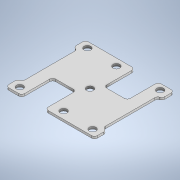
# Autodesk Inventor part: Separador engrenagens
Saved by Autodesk Inventor 2021 (Build 250183000, 183)
## iProperties
Created: 2022-03-26
Part Number: Separador engrenagens
Material: Generic
Document SubType Name: Modeling
Designer: Matheus
Density: 1.04769 g/cm^3
Appearance: Default
Mass: 3.4 g
Surface Area: 49.2715 cm^2
Volume: 3.24524 cm^3
Author: Matheus
Autodesk Inventor part; units mm, degrees
ref_plane "YZ Plane" through (0, 0, 0) normal (1, 0, 0) x (0, 1, 0)
ref_plane "XZ Plane" through (0, 0, 0) normal (0, 1, 0) x (-1, 0, 0)
ref_plane "XY Plane" through (0, 0, 0) normal (0, 0, 1) x (1, 0, 0)
sketch "Sketch1" plane through (0, 0, 0) normal (0, 1, 0) x (-1, 0, 0)
  line L0 (-29.5, 26.5) -> (29.5, 26.5)
  line L1 (29.5, 26.5) -> (29.5, -26.5)
  line L2 (29.5, -26.5) -> (-29.5, -26.5)
  line L3 (-29.5, -26.5) -> (-29.5, 26.5)
  line L4 (-29.5, 26.5) -> (29.5, -26.5) construction
  line L5 (29.5, 26.5) -> (-29.5, -26.5) construction
  point P0 (0, 0)
  dimension "d0" = 59
  dimension "d1" = 53
  constraints: 12 end point, 2 midpoint, 2 parallel, 1 horizontal, 1 perpendicular
  measures "d0" distance of L1.end L2.end
  measures "d1" distance of L0.end L1.end
extrude "Extrusion1" add sketch "Sketch1" along normal blind 1.5
sketch "Sketch2" plane through (0, 1.5, 0) normal (0, 1, 0) x (1, 0, 0)
  line L0 (41.3, 0) -> (-41.3, 0) construction
  line L1 (0, 37.1) -> (0, -37.1) construction
  line L2 (-29.5, 26.5) -> (-29.5, -26.5) construction
  point P0 (0, 0)
  point P1 (-24.25, -22.5)
  point P2 (-24.25, 22.5)
  point P3 (4.15, -21.724)
  point P4 (0, 0)
  point P5 (-4.15, 21.724)
  point P6 (24.25, -22.5)
  point P7 (24.25, 22.5)
  dimension "d5" = 21.724
  dimension "d7" = 45
  dimension "d8" = 24.25
  dimension "d9" = 21.724
  dimension "d19" = 4.15
  dimension "d20" = 4.15
  constraints: 3 symmetric about line, 1 coincident
  measures "d5" distance from line of L0 point (4.15, -21.724)
  measures "d7" distance of point (-24.25, 22.5) point (-24.25, -22.5)
  measures "d8" distance from line of L1 point (-24.25, 22.5)
  measures "d9" vertical distance of point (-4.15, 21.724) point (0, 0)
  measures "d19" distance from line of L1 point (-4.15, 21.724)
  measures "d20" distance from line of L1 point (4.15, -21.724)
hole "Hole1" at (-24.25, 1.5, 22.5) at (-24.25, 1.5, -22.5) at (4.15, 1.5, 21.724) at (0, 1.5, 0) at (-4.15, 1.5, -21.724) at (24.25, 1.5, 22.5) at (24.25, 1.5, -22.5) direction (0, -1, 0) diameter 4.5 depth 1.5
sketch "Sketch3" plane through (0, 1.5, 0) normal (0, 1, 0) x (1, 0, 0)
  line L0 (-41.3, 0) -> (41.3, 0) construction
  line L1 (0, 37.1) -> (0, -37.1) construction
  line L2 (-3.35, -26.5) -> (-19, -26.5)
  line L3 (-19, -26.5) -> (-19, -5.85)
  line L4 (-19, -5.85) -> (-3.35, -5.85)
  line L5 (-3.35, -5.85) -> (-3.35, -26.5)
  line L6 (3.35, 5.85) -> (19, 5.85)
  line L7 (19, 5.85) -> (19, 26.5)
  line L8 (19, 26.5) -> (3.35, 26.5)
  line L9 (3.35, 26.5) -> (3.35, 5.85)
  circle A0 centre (4.15, -21.724) radius 2.25 construction
  line L10 (-29.5, -26.5) -> (29.5, -26.5) construction
  circle A1 centre (-24.25, -22.5) radius 2.25 construction
  line L11 (29.5, 26.5) -> (-29.5, 26.5) construction
  circle A2 centre (24.25, 22.5) radius 2.25 construction
  circle A3 centre (-4.15, 21.724) radius 2.25 construction
  point P0 (0, 0)
  point P1 (-28.5, -26.5)
  point P2 (28.5, -26.5)
  point P3 (28.5, 26.5)
  point P4 (-28.5, 26.5)
  dimension "d21" = 7.5
  dimension "d23" = 5.25
  dimension "d24" = 20.65
  dimension "d25" = 20.65
  dimension "d26" = 7.5
  dimension "d27" = 5.25
  constraints: 16 end point, 4 parallel, 2 collinear, 2 horizontal, 2 perpendicular
  measures "d21" distance from line of L5 A0.centre
  measures "d23" distance from line of L3 A1.centre
  measures "d24" distance between parallel lines of L2 L4
  measures "d25" distance between parallel lines of L6 L8
  measures "d26" distance from line of L9 A3.centre
  measures "d27" distance from line of A2.centre L7
extrude "Extrusion2" cut sketch "Sketch3" against normal up to next
sketch "Sketch5" plane through (0, 1.5, 0) normal (0, 1, 0) x (1, 0, 0)
  line L0 (29.5, -26.5) -> (29.5, 26.5) construction
  line L1 (29.5, 18.5) -> (26.75, 18.5)
  line L2 (26.75, 18.5) -> (26.75, -18.5)
  line L3 (26.75, -18.5) -> (29.5, -18.5)
  line L4 (29.5, -18.5) -> (29.5, 18.5)
  line L5 (-41.3, 0) -> (41.3, 0) construction
  line L6 (0, 37.1) -> (0, -37.1) construction
  line L7 (-29.5, 18.5) -> (-26.75, 18.5)
  line L8 (-26.75, 18.5) -> (-26.75, -18.5)
  line L9 (-26.75, -18.5) -> (-29.5, -18.5)
  line L10 (-29.5, -18.5) -> (-29.5, 18.5)
  point P0 (0, 0)
  dimension "d35" = 37
  dimension "d36" = 2.75
  constraints: 16 end point, 4 symmetric about line, 2 parallel, 1 horizontal, 1 perpendicular, 1 point on line, 1 other
  measures "d35" distance from line of L2.end L1
  measures "d36" distance between parallel lines of L0 L2
extrude "Extrusion4" cut sketch "Sketch5" against normal up to next
fillet "Fillet2" radius 2 20 edges at (-29.5, 0.75, 26.5) (-19, 0.75, 26.5) (-3.35, 0.75, 26.5) (-3.35, 0.75, 5.85) (-19, 0.75, 5.85) (29.5, 0.75, 26.5) (29.5, 0.75, -26.5) (19, 0.75, -26.5) (3.35, 0.75, -26.5) (3.35, 0.75, -5.85) (19, 0.75, -5.85) (-29.5, 0.75, -26.5) (-29.5, 0.75, 18.5) (-26.75, 0.75, 18.5) (-29.5, 0.75, -18.5) (-26.75, 0.75, -18.5) (26.75, 0.75, 18.5) (29.5, 0.75, 18.5) (26.75, 0.75, -18.5) (29.5, 0.75, -18.5)
body "Solid1"
